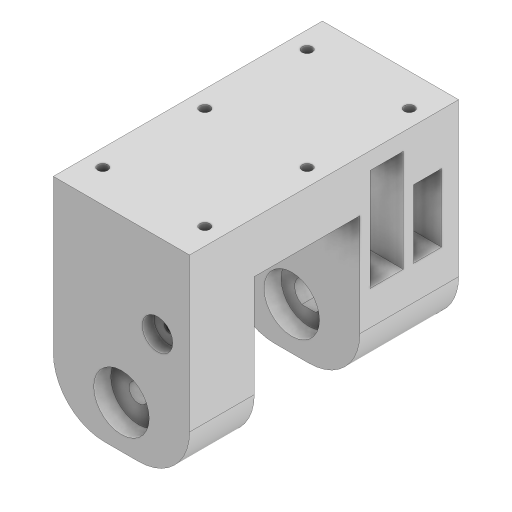
# Autodesk Inventor part: Gimbal_1
Saved by Autodesk Inventor 2023 (Build 270158000, 158)
## iProperties
Created: 2023-10-18
Part Number: Gimbal_1
Material: Generic
Document SubType Name: Modeling
Designer: MVeszpremi
Density: 1 g/cm^3
Appearance: Default
Author: MVeszpremi
Autodesk Inventor part; units mm, degrees
ref_plane "YZ Plane" through (0, 0, 0) normal (1, 0, 0) x (0, 1, 0)
ref_plane "XZ Plane" through (0, 0, 0) normal (0, 1, 0) x (-1, 0, 0)
ref_plane "XY Plane" through (0, 0, 0) normal (0, 0, 1) x (1, 0, 0)
sketch "Sketch1" plane through (0, 0, 0) normal (0, 1, 0) x (-1, 0, 0)
  line L0 (20, 34.5) -> (-20, 34.5)
  line L1 (-20, 34.5) -> (-20, 15.5)
  line L2 (-20, 15.5) -> (20, 15.5)
  line L3 (20, 15.5) -> (20, 34.5)
  line L4 (20, -15.5) -> (-20, -15.5)
  line L5 (-20, -15.5) -> (-20, -44.5)
  line L6 (-20, -44.5) -> (20, -44.5)
  line L7 (20, -44.5) -> (20, -15.5)
  point P0 (0, 0)
  dimension "d0" = 31
  dimension "d1" = 19
  dimension "d2" = 40
  dimension "d3" = 20
  dimension "d4" = 29
  dimension "d50" = 15.5
  constraints: 16 end point, 4 parallel, 2 horizontal, 2 perpendicular, 2 point on line
  measures "d0" distance between parallel lines of L4 L2
  measures "d1" distance of L2.end L0.start
  measures "d2" distance of L0.start L0.end
  measures "d3" distance from line of L3 point (0, 0)
  measures "d4" distance of L6.end L4.start
  measures "d50" distance from line of L2 point (0, 0)
extrude "Extrusion1" add sketch "Sketch1" along normal blind 45
sketch "Sketch2" plane through (20, 0, -44.5) normal (0, 0, -1) x (-1, 0, 0)
  circle A0 centre (20, 12.5) radius 8.125
  line L0 (0, 0) -> (40, 0) projected
  circle A1 centre (20, 12.5) radius 2.75
  point P0 (20, 0)
  point P1 (20, 0)
  dimension "d7" = 16.25
  dimension "d8" = 12.5
  dimension "d9" = 5.5
  constraints: 2 centre point, 1 coincident, 1 midpoint
  measures "d7" diameter of A0
  measures "d8" distance of point (20, 0) A0.centre
  measures "d9" diameter of A1
extrude "Extrusion2" cut sketch "Sketch2" against normal blind 274.75 contours A1
sketch "Sketch3" plane through (0, 45, 0) normal (0, 1, 0) x (1, 0, 0)
  line L0 (20, -34.5) -> (20, -15.5) projected
  line L1 (-20, 44.5) -> (-20, 15.5) projected
  line L2 (20, -34.5) -> (-20, -34.5)
  line L3 (-20, -34.5) -> (-20, 44.5)
  line L4 (-20, 44.5) -> (20, 44.5)
  line L5 (20, 44.5) -> (20, -34.5)
  point P0 (0, 0)
  constraints: 8 end point, 2 parallel, 1 horizontal, 1 perpendicular
extrude "Extrusion3" add sketch "Sketch3" along normal blind 15
sketch "Sketch4" plane through (-20, 0, -44.5) normal (-1, 0, 0) x (0, 0, 1)
  line L0 (5, 55) -> (26, 55)
  line L1 (26, 55) -> (26, 25)
  line L2 (26, 25) -> (5, 25)
  line L3 (5, 25) -> (5, 55)
  line L4 (0, 0) -> (0, 60) projected
  line L5 (29, 0) -> (29, 45) projected
  line L6 (0, 60) -> (79, 60) projected
  line L7 (0, 0) -> (29, 0) projected
  line L8 (13.25, 55) -> (16.25, 55)
  line L9 (16.25, 55) -> (16.25, 25)
  line L10 (16.25, 25) -> (13.25, 25)
  line L11 (13.25, 25) -> (13.25, 55)
  line L12 (5, 55) -> (13.25, 55)
  line L13 (13.25, 45) -> (5, 45)
  point P0 (44.5, 0)
  dimension "d14" = 5
  dimension "d15" = 3
  dimension "d16" = 5
  dimension "d18" = 3
  dimension "d19" = 9.75
  dimension "d45" = 25
  constraints: 20 end point, 6 point on line, 4 parallel, 4 perpendicular, 2 horizontal
  measures "d14" distance between parallel lines of L4 L3
  measures "d15" distance between parallel lines of L5 L1
  measures "d16" distance between parallel lines of L6 L0
  measures "d18" distance between parallel lines of L9 L11
  measures "d19" distance between parallel lines of L1 L9
  measures "d45" distance between parallel lines of L7 L2
extrude "Extrusion4" cut sketch "Sketch4" against normal blind 100 contours L13 L11 L2 L3 | L0 L1 L2 L9
sketch "Sketch5" plane through (20, 0, -44.5) normal (0, 0, -1) x (-1, 0, 0)
  circle A0 centre (20, 12.5) radius 2.75 projected
  circle A1 centre (20, 12.5) radius 4.15
  line L0 (17.9354, 8.9) -> (22.0646, 8.9)
  point P0 (20, 0)
  dimension "d22" = 8.3
  dimension "d24" = 3.6
  constraints: 2 end point, 2 point on circle, 1 centre point, 1 coincident, 1 horizontal
  measures "d22" diameter of A1
  measures "d24" distance from line of L0 A1.centre
extrude "Extrusion5" cut sketch "Sketch5" against normal blind 25 contours A1 L0 picked at (20.1105, 9.19)
sketch "Sketch6" plane through (20, 0, -44.5) normal (0, 0, -1) x (-1, 0, 0)
  line L0 (16.375, 7) -> (23.625, 7)
  line L1 (23.625, 7) -> (23.625, 3.5)
  line L2 (23.625, 3.5) -> (16.375, 3.5)
  line L3 (16.375, 3.5) -> (16.375, 7)
  line L4 (0, 0) -> (40, 0) projected
  circle A0 centre (20, 12.5) radius 2.75 projected
  point P0 (20, 0)
  point P1 (20, 0)
  dimension "d27" = 3.5
  dimension "d28" = 7.25
  dimension "d29" = 3.625
  dimension "d30" = 5.5
  constraints: 8 end point, 2 parallel, 1 horizontal, 1 midpoint, 1 perpendicular
  measures "d27" distance between parallel lines of L2 L0
  measures "d28" distance of L0.start L0.end
  measures "d29" horizontal distance of point (20, 0) L2.end
  measures "d30" distance from line of A0.centre L0
extrude "Extrusion6" cut sketch "Sketch6" against normal blind 23 contours L0 L1 L2 L3
sketch "Sketch7" plane through (0, 0, 0) normal (0, -1, 0) x (1, 0, 0)
  circle A0 centre (0, -37.5) radius 2
  point P0 (0, 0)
  dimension "d33" = 4
  dimension "d34" = 37.5
  constraints: 1 centre point
  measures "d33" diameter of A0
  measures "d34" distance of point (0, 0) A0.centre
extrude "Extrusion7" cut sketch "Sketch7" against normal blind 15.5
sketch "Sketch8" plane through (-20, 0, -15.5) normal (0, 0, 1) x (1, 0, 0)
  circle A0 centre (20, 12.5) radius 2.75 projected
  circle A1 centre (20, 12.5) radius 8.15
  point P0 (20, 0)
  dimension "d37" = 16.3
  constraints: 1 centre point, 1 coincident
  measures "d37" diameter of A1
extrude "Extrusion8" cut sketch "Sketch8" against normal blind 5
sketch "Sketch9" plane through (-20, 0, 34.5) normal (0, 0, 1) x (1, 0, 0)
  circle A0 centre (20, 12.5) radius 2.75 projected
  circle A1 centre (20, 12.5) radius 8.15
  point P0 (20, 0)
  constraints: 1 centre point, 1 coincident
extrude "Extrusion9" cut sketch "Sketch9" against normal blind 5
sketch "Sketch10" plane through (20, 0, 15.5) normal (0, 0, -1) x (-1, 0, 0)
  circle A0 centre (20, 12.5) radius 2.75 projected
  circle A1 centre (20, 12.5) radius 8.15
  point P0 (20, 0)
  constraints: 1 centre point, 1 coincident
extrude "Extrusion10" cut sketch "Sketch10" against normal blind 5
fillet "Fillet1" radius 15 4 edges at (-20, 0, -30) (-20, 0, 25) (20, 0, 25) (20, 0, -30)
sketch "Sketch11" plane through (0, 60, 0) normal (0, 1, 0) x (1, 0, 0)
  line L0 (-15, -25) -> (15, -25)
  line L1 (15, -25) -> (15, 35)
  line L2 (15, 35) -> (-15, 35)
  line L3 (-15, 35) -> (-15, -25)
  circle A0 centre (-15, -25) radius 1.5
  circle A1 centre (-15, 35) radius 1.5
  circle A2 centre (15, 35) radius 1.5
  circle A3 centre (15, -25) radius 1.5
  circle A4 centre (-15, 5) radius 1.5
  circle A5 centre (15, 5) radius 1.5
  point P0 (0, 0)
  dimension "d46" = 60
  dimension "d47" = 30
  dimension "d48" = 15
  dimension "d49" = 25
  dimension "d51" = 3
  dimension "d52" = 3
  dimension "d53" = 3
  dimension "d54" = 3
  dimension "d55" = 3
  dimension "d56" = 3
  constraints: 8 end point, 6 centre point, 4 coincident, 2 midpoint, 2 parallel, 1 horizontal, 1 perpendicular
  measures "d46" distance of L2.end L0.start
  measures "d47" distance of L0.start L0.end
  measures "d48" distance from line of L3 point (0, 0)
  measures "d49" distance from line of L0 point (0, 0)
  measures "d51" diameter of A0
  measures "d52" diameter of A1
  measures "d53" diameter of A2
  measures "d54" diameter of A3
  measures "d55" diameter of A4
  measures "d56" diameter of A5
extrude "Extrusion11" cut sketch "Sketch11" against normal blind 15 contours L3 A0 L0 | L0 A0 L3 | A3 L1 L0 | L0 L1 A3 | A4 L3 | L3 A4 | A5 L1 | L1 A5 | A1 L2 L3 | L3 L2 A1 | A2 L2 L1 | L1 L2 A2
sketch "Sketch12" plane through (20, 60, -44.5) normal (0, 0, -1) x (-1, 0, 0)
  arc A0 (22.0646, -51.1) -> (17.9354, -51.1) centre (20, -47.5) ccw projected
  circle A1 centre (20, -47.5) radius 4.15
  point P0 (20, -60)
  constraints: 1 centre point, 1 coincident
extrude "Extrusion12" cut sketch "Sketch12" against normal blind 2
sketch "Sketch13" plane through (20, 60, -44.5) normal (0, 0, -1) x (-1, 0, 0)
  arc A0 (22.0646, -51.1) -> (17.9354, -51.1) centre (20, -47.5) ccw projected
  circle A1 centre (20, -47.5) radius 10
  line L0 (20, -37.5) -> (40, -37.5)
  line L1 (40, -37.5) -> (0, -37.5)
  line L2 (0, -45) -> (0, 0) projected
  circle A2 centre (20, -47.5) radius 4.15 projected
  arc A3 (0, -45) -> (15, -60) centre (15, -45) ccw projected
  line L3 (15, -60) -> (25, -60) projected
  arc A4 (25, -60) -> (40, -45) centre (25, -45) ccw projected
  line L4 (40, -45) -> (40, 0) projected
  line L5 (0, 0) -> (40, 0) projected
  line L6 (0, -45) -> (0, 0) projected
  line L7 (23.625, -53) -> (23.625, -56.5) projected
  line L8 (23.625, -56.5) -> (16.375, -56.5) projected
  line L9 (16.375, -56.5) -> (16.375, -53) projected
  line L10 (16.375, -53) -> (23.625, -53) projected
  circle A5 centre (20, -47.5) radius 18
  point P0 (20, -60)
  point P1 (20, -37.5)
  point P2 (20, -37.5)
  point P3 (3.4436, -54.5629)
  point P4 (34.9666, -37.5)
  point P5 (36.5564, -54.5629)
  dimension "d61" = 20
  dimension "d64" = 36
  constraints: 4 end point, 2 coincident, 2 point on line, 1 centre point, 1 horizontal, 3 other
  measures "d64" diameter of A5
extrude "Extrusion13" cut sketch "Sketch13" against normal blind 1.5 contours A2 A0 | L0 A5 A4 L3 A3 L1 | L1 A5 L0 | L7 L8 L9 L10
sketch "Sketch14" plane through (-20, 60, 34.5) normal (0, 0, 1) x (1, 0, 0)
  circle A0 centre (30.5655, -24.8423) radius 4.5
  circle A1 centre (20, -47.5) radius 2.75 projected
  circle A2 centre (30.5655, -24.8423) radius 1.5
  line L0 (20, -47.5) -> (20, 0.1242)
  line L1 (20, 0.1242) -> (20, -47.5)
  line L2 (30.5655, -24.8423) -> (20, -47.5)
  point P0 (20, -60)
  dimension "d65" = 25
  dimension "d66" = 9
  dimension "d67" = 3
  dimension "d72" = 25
  constraints: 6 end point, 2 centre point, 1 coincident, 1 collinear, 1 vertical
  measures "d65" distance of A0.centre L0.start
  measures "d66" diameter of A0
  measures "d67" diameter of A2
  measures "d72" angle of L2 L0
extrude "Extrusion14" cut sketch "Sketch14" against normal blind 10 contours A2
extrude "Extrusion15" cut sketch "Sketch14" against normal blind 3.5 contours A0
body "Solid1"
